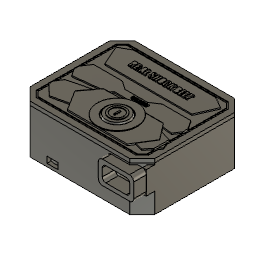
device_case (Autodesk Fusion 360 design; units mm, degrees)
part number: 2026-05-29-19-24-18-307
part number: 2026-05-29-19-24-19-033
part number: 2026-05-29-19-24-19-686
part number: 2026-05-29-19-24-22-511
part number: 2026-05-29-19-24-23-032
Autodesk Fusion 360 part; units mm, degrees
(part 1 of 2)
ref_plane "作業平面1" through (0, 0, 0) normal (0, 0, 1) x (1, 0, 0) in component "CASE_BASE_print"
sketch "スケッチ1" plane through (0, 0, 0) normal (0, 0, 1) x (1, 0, 0) in component "CASE_BASE_print"
  line L0 (-40, -42) -> (40, -42)
  line L1 (40, -42) -> (50, -32)
  line L2 (50, -32) -> (50, 32)
  line L3 (50, 32) -> (40, 42)
  line L4 (40, 42) -> (-40, 42)
  line L5 (-40, 42) -> (-50, 32)
  line L6 (-50, 32) -> (-50, -32)
  line L7 (-50, -32) -> (-40, -42)
extrude "押し出し1" add sketch "スケッチ1" along normal blind 36 makes body 1 in component "CASE_BASE_print"
ref_plane "作業平面2" through (0, 0, 2.4) normal (0, 0, 1) x (1, 0, 0) in component "CASE_BASE_print"
sketch "スケッチ2" plane through (0, 0, 2.4) normal (0, 0, 1) x (1, 0, 0) in component "CASE_BASE_print"
  line L0 (-40, -39.6) -> (40, -39.6)
  line L1 (40, -39.6) -> (47.6, -32)
  line L2 (47.6, -32) -> (47.6, 32)
  line L3 (47.6, 32) -> (40, 39.6)
  line L4 (40, 39.6) -> (-40, 39.6)
  line L5 (-40, 39.6) -> (-47.6, 32)
  line L6 (-47.6, 32) -> (-47.6, -32)
  line L7 (-47.6, -32) -> (-40, -39.6)
extrude "押し出し2" add sketch "スケッチ2" along normal blind 34.1 separate body makes body 2 in component "CASE_BASE_print"
ref_plane "作業平面3" through (0, 0, -0.5) normal (0, 0, 1) x (1, 0, 0) in component "CASE_BASE_print"
sketch "スケッチ3" plane through (0, 0, -0.5) normal (0, 0, 1) x (1, 0, 0) in component "CASE_BASE_print"
  circle A0 centre (-22, -14) radius 25.175
extrude "押し出し3" add sketch "スケッチ3" along normal blind 7.5 separate body makes body 3 in component "CASE_BASE_print"
combine "結合1" operation cut target body 1 tool bodies 2 3 in component "CASE_BASE_print"
ref_plane "作業平面4" through (0, 0, 0) normal (0, 0, 1) x (1, 0, 0) in component "CASE_BASE_print"
sketch "スケッチ4" plane through (0, 0, 0) normal (0, 0, 1) x (1, 0, 0) in component "CASE_BASE_print"
  circle A0 centre (-22, -14) radius 27.375
extrude "押し出し4" add sketch "スケッチ4" along normal blind 6.2 separate body makes body 4 in component "CASE_BASE_print"
ref_plane "作業平面5" through (0, 0, -0.2) normal (0, 0, 1) x (1, 0, 0) in component "CASE_BASE_print"
sketch "スケッチ5" plane through (0, 0, -0.2) normal (0, 0, 1) x (1, 0, 0) in component "CASE_BASE_print"
  circle A0 centre (-22, -14) radius 25.175
extrude "押し出し5" add sketch "スケッチ5" along normal blind 6.8 separate body makes body 5 in component "CASE_BASE_print"
combine "結合2" operation cut target body 4 tool bodies 5 in component "CASE_BASE_print"
combine "結合3" operation add target body 1 tool bodies 4 in component "CASE_BASE_print"
ref_plane "作業平面6" through (0, 0, 2.5) normal (0, 0, 1) x (1, 0, 0) in component "CASE_BASE_print"
sketch "スケッチ6" plane through (0, 0, 2.5) normal (0, 0, 1) x (1, 0, 0) in component "CASE_BASE_print"
  line L0 (-26.5, -42.5) -> (-17.5, -42.5)
  line L1 (-17.5, -42.5) -> (-17.5, -32)
  line L2 (-17.5, -32) -> (-26.5, -32)
  line L3 (-26.5, -32) -> (-26.5, -42.5)
extrude "押し出し6" add sketch "スケッチ6" along normal blind 5 separate body makes body 6 in component "CASE_BASE_print"
ref_plane "作業平面7" through (0, -42.7, 0) normal (0, 1, 0) x (0, 0, 1) in component "CASE_BASE_print"
sketch "スケッチ7" plane through (0, -42.7, 0) normal (0, 1, 0) x (1, 0, 0) in component "CASE_BASE_print"
  line L0 (27.8, 19.5) -> (44.2, 19.5)
  arc A0 (44.2, 19.5) -> (47, 22.3) centre (44.2, 22.3) ccw
  line L1 (47, 22.3) -> (47, 28.7)
  arc A1 (47, 28.7) -> (44.2, 31.5) centre (44.2, 28.7) ccw
  line L2 (44.2, 31.5) -> (27.8, 31.5)
  arc A2 (27.8, 31.5) -> (25, 28.7) centre (27.8, 28.7) ccw
  line L3 (25, 28.7) -> (25, 22.3)
  arc A3 (25, 22.3) -> (27.8, 19.5) centre (27.8, 22.3) ccw
extrude "押し出し7" add sketch "スケッチ7" along normal blind 7.1 separate body makes body 7 in component "CASE_BASE_print"
move_body "移動1" bodies 7 to x (1, 0, 0) y (0, 1, 0) z (0, 0, 1) at (0, 0, 51) in component "CASE_BASE_print"
combine "結合4" operation cut target body 1 tool bodies 6 7 in component "CASE_BASE_print"
ref_plane "作業平面8" through (0, -49, 0) normal (0, 1, 0) x (0, 0, 1) in component "CASE_BASE_print"
sketch "スケッチ8" plane through (0, -49, 0) normal (0, 1, 0) x (1, 0, 0) in component "CASE_BASE_print"
  line L0 (25.2, 16.3) -> (46.8, 16.3)
  arc A0 (46.8, 16.3) -> (50.2, 19.7) centre (46.8, 19.7) ccw
  line L1 (50.2, 19.7) -> (50.2, 31.3)
  arc A1 (50.2, 31.3) -> (46.8, 34.7) centre (46.8, 31.3) ccw
  line L2 (46.8, 34.7) -> (25.2, 34.7)
  arc A2 (25.2, 34.7) -> (21.8, 31.3) centre (25.2, 31.3) ccw
  line L3 (21.8, 31.3) -> (21.8, 19.7)
  arc A3 (21.8, 19.7) -> (25.2, 16.3) centre (25.2, 19.7) ccw
extrude "押し出し8" add sketch "スケッチ8" along normal blind 10.2 separate body makes body 8 in component "CASE_BASE_print"
move_body "移動2" bodies 8 to x (1, 0, 0) y (0, 1, 0) z (0, 0, 1) at (0, 0, 51) in component "CASE_BASE_print"
ref_plane "作業平面9" through (0, -49.2, 0) normal (0, 1, 0) x (0, 0, 1) in component "CASE_BASE_print"
sketch "スケッチ9" plane through (0, -49.2, 0) normal (0, 1, 0) x (1, 0, 0) in component "CASE_BASE_print"
  line L0 (27.8, 19.5) -> (44.2, 19.5)
  arc A0 (44.2, 19.5) -> (47, 22.3) centre (44.2, 22.3) ccw
  line L1 (47, 22.3) -> (47, 28.7)
  arc A1 (47, 28.7) -> (44.2, 31.5) centre (44.2, 28.7) ccw
  line L2 (44.2, 31.5) -> (27.8, 31.5)
  arc A2 (27.8, 31.5) -> (25, 28.7) centre (27.8, 28.7) ccw
  line L3 (25, 28.7) -> (25, 22.3)
  arc A3 (25, 22.3) -> (27.8, 19.5) centre (27.8, 22.3) ccw
extrude "押し出し9" add sketch "スケッチ9" along normal blind 10.6 separate body makes body 9 in component "CASE_BASE_print"
move_body "移動3" bodies 9 to x (1, 0, 0) y (0, 1, 0) z (0, 0, 1) at (0, 0, 51) in component "CASE_BASE_print"
combine "結合5" operation cut target body 8 tool bodies 9 in component "CASE_BASE_print"
combine "結合6" operation add target body 1 tool bodies 8 in component "CASE_BASE_print"
ref_plane "作業平面10" through (0, 0, 16.3) normal (0, 0, 1) x (1, 0, 0) in component "CASE_BASE_print"
sketch "スケッチ10" plane through (0, 0, 16.3) normal (0, 0, 1) x (1, 0, 0) in component "CASE_BASE_print"
  line L0 (47, -38.8) -> (50, -38.8)
  line L1 (50, -38.8) -> (50, -32)
  line L2 (50, -32) -> (47, -35)
  line L3 (47, -35) -> (47, -38.8)
extrude "押し出し10" add sketch "スケッチ10" along normal blind 18.4 separate body makes body 10 in component "CASE_BASE_print"
combine "結合7" operation add target body 1 tool bodies 10 in component "CASE_BASE_print"
ref_plane "作業平面11" through (0, 0, 2.4) normal (0, 0, 1) x (1, 0, 0) in component "CASE_BASE_print"
sketch "スケッチ11" plane through (0, 0, 2.4) normal (0, 0, 1) x (1, 0, 0) in component "CASE_BASE_print"
  circle A0 centre (12, -24) radius 2.9
extrude "押し出し11" add sketch "スケッチ11" along normal blind 15.1 separate body makes body 11 in component "CASE_BASE_print"
ref_plane "作業平面12" through (0, 0, 2.2) normal (0, 0, 1) x (1, 0, 0) in component "CASE_BASE_print"
sketch "スケッチ12" plane through (0, 0, 2.2) normal (0, 0, 1) x (1, 0, 0) in component "CASE_BASE_print"
  circle A0 centre (12, -24) radius 1.1
extrude "押し出し12" add sketch "スケッチ12" along normal blind 15.7 separate body makes body 12 in component "CASE_BASE_print"
combine "結合8" operation cut target body 11 tool bodies 12 in component "CASE_BASE_print"
ref_plane "作業平面13" through (0, 0, 2.4) normal (0, 0, 1) x (1, 0, 0) in component "CASE_BASE_print"
sketch "スケッチ13" plane through (0, 0, 2.4) normal (0, 0, 1) x (1, 0, 0) in component "CASE_BASE_print"
  circle A0 centre (42, -24) radius 2.9
extrude "押し出し13" add sketch "スケッチ13" along normal blind 15.1 separate body makes body 13 in component "CASE_BASE_print"
ref_plane "作業平面14" through (0, 0, 2.2) normal (0, 0, 1) x (1, 0, 0) in component "CASE_BASE_print"
sketch "スケッチ14" plane through (0, 0, 2.2) normal (0, 0, 1) x (1, 0, 0) in component "CASE_BASE_print"
  circle A0 centre (42, -24) radius 1.1
extrude "押し出し14" add sketch "スケッチ14" along normal blind 15.7 separate body makes body 14 in component "CASE_BASE_print"
combine "結合9" operation cut target body 13 tool bodies 14 in component "CASE_BASE_print"
ref_plane "作業平面15" through (0, 0, 2.4) normal (0, 0, 1) x (1, 0, 0) in component "CASE_BASE_print"
sketch "スケッチ15" plane through (0, 0, 2.4) normal (0, 0, 1) x (1, 0, 0) in component "CASE_BASE_print"
  circle A0 centre (-2, 28) radius 2.9
extrude "押し出し15" add sketch "スケッチ15" along normal blind 15.1 separate body makes body 15 in component "CASE_BASE_print"
ref_plane "作業平面16" through (0, 0, 2.2) normal (0, 0, 1) x (1, 0, 0) in component "CASE_BASE_print"
sketch "スケッチ16" plane through (0, 0, 2.2) normal (0, 0, 1) x (1, 0, 0) in component "CASE_BASE_print"
  circle A0 centre (-2, 28) radius 1.1
extrude "押し出し16" add sketch "スケッチ16" along normal blind 15.7 separate body makes body 16 in component "CASE_BASE_print"
combine "結合10" operation cut target body 15 tool bodies 16 in component "CASE_BASE_print"
ref_plane "作業平面17" through (0, 0, 2.4) normal (0, 0, 1) x (1, 0, 0) in component "CASE_BASE_print"
sketch "スケッチ17" plane through (0, 0, 2.4) normal (0, 0, 1) x (1, 0, 0) in component "CASE_BASE_print"
  circle A0 centre (42, 28) radius 2.9
extrude "押し出し17" add sketch "スケッチ17" along normal blind 15.1 separate body makes body 17 in component "CASE_BASE_print"
ref_plane "作業平面18" through (0, 0, 2.2) normal (0, 0, 1) x (1, 0, 0) in component "CASE_BASE_print"
sketch "スケッチ18" plane through (0, 0, 2.2) normal (0, 0, 1) x (1, 0, 0) in component "CASE_BASE_print"
  circle A0 centre (42, 28) radius 1.1
extrude "押し出し18" add sketch "スケッチ18" along normal blind 15.7 separate body makes body 18 in component "CASE_BASE_print"
combine "結合11" operation cut target body 17 tool bodies 18 in component "CASE_BASE_print"
combine "結合12" operation add target body 1 tool bodies 11 13 15 17 in component "CASE_BASE_print"
ref_plane "作業平面1" through (0, 0, 36) normal (0, 0, 1) x (1, 0, 0) in component "CASE_LID_print"
sketch "スケッチ1 (2)" plane through (0, 0, 36) normal (0, 0, 1) x (1, 0, 0) in component "CASE_LID_print"
  line L0 (-40, -42) -> (40, -42)
  line L1 (40, -42) -> (50, -32)
  line L2 (50, -32) -> (50, 32)
  line L3 (50, 32) -> (40, 42)
  line L4 (40, 42) -> (-40, 42)
  line L5 (-40, 42) -> (-50, 32)
  line L6 (-50, 32) -> (-50, -32)
  line L7 (-50, -32) -> (-40, -42)
extrude "押し出し1'" add sketch "スケッチ1 (2)" along normal blind 3 separate body makes body 19 in component "CASE_LID_print"
ref_plane "作業平面2" through (0, 0, 33) normal (0, 0, 1) x (1, 0, 0) in component "CASE_LID_print"
sketch "スケッチ2 (2)" plane through (0, 0, 33) normal (0, 0, 1) x (1, 0, 0) in component "CASE_LID_print"
  line L0 (-40, -39.25) -> (40, -39.25)
  line L1 (40, -39.25) -> (47.25, -32)
  line L2 (47.25, -32) -> (47.25, 32)
  line L3 (47.25, 32) -> (40, 39.25)
  line L4 (40, 39.25) -> (-40, 39.25)
  line L5 (-40, 39.25) -> (-47.25, 32)
  line L6 (-47.25, 32) -> (-47.25, -32)
  line L7 (-47.25, -32) -> (-40, -39.25)
extrude "押し出し2'" add sketch "スケッチ2 (2)" along normal blind 3 separate body makes body 20 in component "CASE_LID_print"
ref_plane "作業平面3" through (0, 0, 32.8) normal (0, 0, 1) x (1, 0, 0) in component "CASE_LID_print"
sketch "スケッチ3 (2)" plane through (0, 0, 32.8) normal (0, 0, 1) x (1, 0, 0) in component "CASE_LID_print"
  line L0 (-40, -37.45) -> (40, -37.45)
  line L1 (40, -37.45) -> (45.45, -32)
  line L2 (45.45, -32) -> (45.45, 32)
  line L3 (45.45, 32) -> (40, 37.45)
  line L4 (40, 37.45) -> (-40, 37.45)
  line L5 (-40, 37.45) -> (-45.45, 32)
  line L6 (-45.45, 32) -> (-45.45, -32)
  line L7 (-45.45, -32) -> (-40, -37.45)
extrude "押し出し3'" add sketch "スケッチ3 (2)" along normal blind 3.4 separate body makes body 21 in component "CASE_LID_print"
combine "結合1'" operation cut target body 20 tool bodies 21 in component "CASE_LID_print"
combine "結合2'" operation add target body 19 tool bodies 20 in component "CASE_LID_print"
ref_plane "作業平面4" through (0, 0, 32.7) normal (0, 0, 1) x (1, 0, 0) in component "CASE_LID_print"
sketch "スケッチ4 (2)" plane through (0, 0, 32.7) normal (0, 0, 1) x (1, 0, 0) in component "CASE_LID_print"
  circle A0 centre (6, -18) radius 5.25
extrude "押し出し4'" add sketch "スケッチ4 (2)" along normal blind 6.6 separate body makes body 22 in component "CASE_LID_print"
ref_plane "作業平面5" through (0, 0, 35) normal (0, 0, 1) x (1, 0, 0) in component "CASE_LID_print"
sketch "スケッチ5 (2)" plane through (0, 0, 35) normal (0, 0, 1) x (1, 0, 0) in component "CASE_LID_print"
  circle A0 centre (6, -18) radius 9.9
extrude "押し出し5'" add sketch "スケッチ5 (2)" along normal blind 4.3 separate body makes body 23 in component "CASE_LID_print"
combine "結合3'" operation cut target body 19 tool bodies 22 23 in component "CASE_LID_print"
ref_plane "作業平面6" through (0, 0, 26) normal (0, 0, 1) x (1, 0, 0) in component "CASE_LID_print"
sketch "スケッチ6 (2)" plane through (0, 0, 26) normal (0, 0, 1) x (1, 0, 0) in component "CASE_LID_print"
  circle A0 centre (6, -18) radius 11.5
extrude "押し出し6'" add sketch "スケッチ6 (2)" along normal blind 10.6 separate body makes body 24 in component "CASE_LID_print"
ref_plane "作業平面7" through (0, 0, 25.8) normal (0, 0, 1) x (1, 0, 0) in component "CASE_LID_print"
sketch "スケッチ7 (2)" plane through (0, 0, 25.8) normal (0, 0, 1) x (1, 0, 0) in component "CASE_LID_print"
  circle A0 centre (6, -18) radius 5.25
extrude "押し出し7'" add sketch "スケッチ7 (2)" along normal blind 11.1 separate body makes body 25 in component "CASE_LID_print"
combine "結合4'" operation cut target body 24 tool bodies 25 in component "CASE_LID_print"
combine "結合5'" operation add target body 19 tool bodies 24 in component "CASE_LID_print"
ref_plane "作業平面8" through (0, 0, 38.95) normal (0, 0, 1) x (1, 0, 0) in component "CASE_LID_print"
sketch "スケッチ8 (2)" plane through (0, 0, 38.95) normal (0, 0, 1) x (1, 0, 0) in component "CASE_LID_print"
  line L0 (-42, 29) -> (-33, 34)
  line L1 (-33, 34) -> (33, 34)
  line L2 (33, 34) -> (42, 29)
  line L3 (42, 29) -> (35, 13)
  line L4 (35, 13) -> (-35, 13)
  line L5 (-35, 13) -> (-42, 29)
extrude "押し出し8'" add sketch "スケッチ8 (2)" along normal blind 1 separate body makes body 26 in component "CASE_LID_print"
ref_plane "作業平面9" through (0, 0, 38.95) normal (0, 0, 1) x (1, 0, 0) in component "CASE_LID_print"
sketch "スケッチ9 (2)" plane through (0, 0, 38.95) normal (0, 0, 1) x (1, 0, 0) in component "CASE_LID_print"
  line L0 (-39, 8) -> (-16, 8)
  line L1 (-16, 8) -> (-8, 2.5)
  line L2 (-8, 2.5) -> (-14, -5.5)
  line L3 (-14, -5.5) -> (-40, -8.5)
  line L4 (-40, -8.5) -> (-45, -1)
  line L5 (-45, -1) -> (-39, 8)
extrude "押し出し9'" add sketch "スケッチ9 (2)" along normal blind 1 separate body makes body 27 in component "CASE_LID_print"
ref_plane "作業平面10" through (0, 0, 38.95) normal (0, 0, 1) x (1, 0, 0) in component "CASE_LID_print"
sketch "スケッチ10 (2)" plane through (0, 0, 38.95) normal (0, 0, 1) x (1, 0, 0) in component "CASE_LID_print"
  line L0 (39, 8) -> (16, 8)
  line L1 (16, 8) -> (8, 2.5)
  line L2 (8, 2.5) -> (14, -5.5)
  line L3 (14, -5.5) -> (40, -8.5)
  line L4 (40, -8.5) -> (45, -1)
  line L5 (45, -1) -> (39, 8)
extrude "押し出し10'" add sketch "スケッチ10 (2)" along normal blind 1 separate body makes body 28 in component "CASE_LID_print"
ref_plane "作業平面11" through (0, 0, 38.95) normal (0, 0, 1) x (1, 0, 0) in component "CASE_LID_print"
sketch "スケッチ11 (2)" plane through (0, 0, 38.95) normal (0, 0, 1) x (1, 0, 0) in component "CASE_LID_print"
  line L0 (-40, -14) -> (-20, -9)
  line L1 (-20, -9) -> (-7, -14)
  line L2 (-7, -14) -> (-15, -27)
  line L3 (-15, -27) -> (-35, -31.5)
  line L4 (-35, -31.5) -> (-45, -22)
  line L5 (-45, -22) -> (-40, -14)
extrude "押し出し11'" add sketch "スケッチ11 (2)" along normal blind 1 separate body makes body 29 in component "CASE_LID_print"
ref_plane "作業平面12" through (0, 0, 38.95) normal (0, 0, 1) x (1, 0, 0) in component "CASE_LID_print"
sketch "スケッチ12 (2)" plane through (0, 0, 38.95) normal (0, 0, 1) x (1, 0, 0) in component "CASE_LID_print"
  line L0 (44, -14) -> (26, -9)
  line L1 (26, -9) -> (13, -14)
  line L2 (13, -14) -> (21, -27)
  line L3 (21, -27) -> (39, -31.5)
  line L4 (39, -31.5) -> (47, -22)
  line L5 (47, -22) -> (44, -14)
extrude "押し出し12'" add sketch "スケッチ12 (2)" along normal blind 1 separate body makes body 30 in component "CASE_LID_print"
ref_plane "作業平面13" through (0, 0, 38.95) normal (0, 0, 1) x (1, 0, 0) in component "CASE_LID_print"
sketch "スケッチ13 (2)" plane through (0, 0, 38.95) normal (0, 0, 1) x (1, 0, 0) in component "CASE_LID_print"
  line L0 (-18, -5) -> (30, -5)
  line L1 (30, -5) -> (40, -18)
  line L2 (40, -18) -> (30, -34)
  line L3 (30, -34) -> (-18, -34)
  line L4 (-18, -34) -> (-28, -18)
  line L5 (-28, -18) -> (-18, -5)
extrude "押し出し13'" add sketch "スケッチ13 (2)" along normal blind 1.2 separate body makes body 31 in component "CASE_LID_print"
ref_plane "作業平面14" through (0, 0, 38.95) normal (0, 0, 1) x (1, 0, 0) in component "CASE_LID_print"
sketch "スケッチ14 (2)" plane through (0, 0, 38.95) normal (0, 0, 1) x (1, 0, 0) in component "CASE_LID_print"
  line L0 (-13, -2.6) -> (25, -2.6)
  line L1 (25, -2.6) -> (28, 0.5)
  line L2 (28, 0.5) -> (24, 3.3)
  line L3 (24, 3.3) -> (-12, 3.3)
  line L4 (-12, 3.3) -> (-16, 0.5)
  line L5 (-16, 0.5) -> (-13, -2.6)
extrude "押し出し14'" add sketch "スケッチ14 (2)" along normal blind 1 separate body makes body 32 in component "CASE_LID_print"
combine "結合6'" operation add target body 19 tool bodies 26 27 28 29 30 31 32 in component "CASE_LID_print"
ref_plane "作業平面15" through (0, 0, 39.9) normal (0, 0, 1) x (1, 0, 0) in component "CASE_LID_print"
sketch "スケッチ15 (2)" plane through (0, 0, 39.9) normal (0, 0, 1) x (1, 0, 0) in component "CASE_LID_print"
  line L0 (0.01, 25.6699) -> (1.0286, 25.6699)
  spline S0 degree 3 poles (1.0286, 25.6699) (1.3136, 25.6712) (1.7747, 25.6732) (2.2316, 25.6139) (2.406, 25.5913) knots 0 0 0 0 0.085386 0.138098 0.138098 0.138098 0.138098
  spline S1 degree 3 poles (2.406, 25.5913) (2.5217, 25.5539) (2.7574, 25.4777) (2.9141, 25.2857) (2.9939, 25.188) knots 0 0 0 0 0.03568 0.072659 0.072659 0.072659 0.072659
  spline S2 degree 3 poles (2.9939, 25.188) (3.0603, 25.0509) (3.2169, 24.7278) (3.2207, 24.367) (3.2229, 24.1592) knots 0 0 0 0 0.045177 0.106541 0.106541 0.106541 0.106541
  spline S3 degree 3 poles (3.2229, 24.1592) (3.2243, 23.9759) (3.2267, 23.6744) (3.1086, 23.399) (3.0622, 23.291) knots 0 0 0 0 0.054153 0.089108 0.089108 0.089108 0.089108
  spline S4 degree 3 poles (3.0622, 23.291) (2.9864, 23.2238) (2.8077, 23.0654) (2.568, 23.0394) (2.4299, 23.0244) knots 0 0 0 0 0.029736 0.070118 0.070118 0.070118 0.070118
  spline S5 degree 3 poles (2.4299, 23.0244) (2.5541, 22.9928) (2.7668, 22.9388) (2.9344, 22.7989) (3.0041, 22.7407) knots 0 0 0 0 0.037806 0.064758 0.064758 0.064758 0.064758
  spline S6 degree 3 poles (3.0041, 22.7407) (3.0476, 22.6858) (3.1264, 22.5863) (3.1671, 22.4664) (3.1853, 22.4126) knots 0 0 0 0 0.020812 0.037727 0.037727 0.037727 0.037727
  spline S7 degree 3 poles (3.1853, 22.4126) (3.196, 22.3201) (3.2275, 22.0489) (3.2247, 21.7757) (3.2229, 21.5957) knots 0 0 0 0 0.027914 0.08184 0.08184 0.08184 0.08184
  line L1 (3.2229, 21.5957) -> (3.2229, 20.1362)
  line L2 (3.2229, 20.1362) -> (1.8865, 20.1362)
  line L3 (1.8865, 20.1362) -> (1.8865, 21.9751)
  spline S8 degree 3 poles (1.8865, 21.9751) (1.8891, 22.0964) (1.8931, 22.2844) (1.8352, 22.4623) (1.8147, 22.5254) knots 0 0 0 0 0.036019 0.05582 0.05582 0.05582 0.05582
  spline S9 degree 3 poles (1.8147, 22.5254) (1.7742, 22.5559) (1.668, 22.6359) (1.5327, 22.6331) (1.449, 22.6313) knots 0 0 0 0 0.014864 0.039021 0.039021 0.039021 0.039021
  line L4 (1.449, 22.6313) -> (1.449, 20.1362)
  line L5 (1.449, 20.1362) -> (0.01, 20.1362)
  line L6 (0.01, 20.1362) -> (0.01, 25.6699)
  line L7 (1.449, 24.7231) -> (1.449, 23.4927)
  spline S10 degree 3 poles (1.449, 23.4927) (1.5188, 23.4926) (1.6363, 23.4925) (1.7438, 23.5388) (1.7873, 23.5576) knots 0 0 0 0 0.020657 0.034769 0.034769 0.034769 0.034769
  spline S11 degree 3 poles (1.7873, 23.5576) (1.8157, 23.6041) (1.8956, 23.7352) (1.8901, 23.8911) (1.8865, 23.9917) knots 0 0 0 0 0.01609 0.045334 0.045334 0.045334 0.045334
  line L8 (1.8865, 23.9917) -> (1.8865, 24.2959)
  spline S12 degree 3 poles (1.8865, 24.2959) (1.8869, 24.3712) (1.8875, 24.4968) (1.8184, 24.5999) (1.7908, 24.6411) knots 0 0 0 0 0.021921 0.036536 0.036536 0.036536 0.036536
  spline S13 degree 3 poles (1.7908, 24.6411) (1.7478, 24.6648) (1.6423, 24.723) (1.5209, 24.7231) (1.449, 24.7231) knots 0 0 0 0 0.014526 0.035647 0.035647 0.035647 0.035647
  line L9 (3.78, 25.6699) -> (6.1794, 25.6699)
  line L10 (6.1794, 25.6699) -> (6.1794, 24.5625)
  line L11 (6.1794, 24.5625) -> (5.219, 24.5625)
  line L12 (5.219, 24.5625) -> (5.219, 23.5132)
  line L13 (5.219, 23.5132) -> (6.1179, 23.5132)
  line L14 (6.1179, 23.5132) -> (6.1179, 22.4604)
  line L15 (6.1179, 22.4604) -> (5.219, 22.4604)
  line L16 (5.219, 22.4604) -> (5.219, 21.2436)
  line L17 (5.219, 21.2436) -> (6.2751, 21.2436)
  line L18 (6.2751, 21.2436) -> (6.2751, 20.1362)
  line L19 (6.2751, 20.1362) -> (3.78, 20.1362)
  line L20 (3.78, 20.1362) -> (3.78, 25.6699)
  line L21 (7.6902, 23.7388) -> (7.6902, 22.6142)
  line L22 (7.6902, 22.6142) -> (6.6477, 22.6142)
  line L23 (6.6477, 22.6142) -> (6.6477, 23.7388)
  line L24 (6.6477, 23.7388) -> (7.6902, 23.7388)
  line L25 (7.6902, 21.2641) -> (7.6902, 20.1362)
  line L26 (7.6902, 20.1362) -> (6.6477, 20.1362)
  line L27 (6.6477, 20.1362) -> (6.6477, 21.2641)
  line L28 (6.6477, 21.2641) -> (7.6902, 21.2641)
  line L29 (10.5886, 25.6699) -> (11.4123, 20.1362)
  line L30 (11.4123, 20.1362) -> (9.9392, 20.1362)
  line L31 (9.9392, 20.1362) -> (9.8674, 21.1308)
  line L32 (9.8674, 21.1308) -> (9.3513, 21.1308)
  line L33 (9.3513, 21.1308) -> (9.2659, 20.1362)
  line L34 (9.2659, 20.1362) -> (7.7756, 20.1362)
  line L35 (7.7756, 20.1362) -> (8.5071, 25.6699)
  line L36 (8.5071, 25.6699) -> (10.5886, 25.6699)
  spline S14 degree 3 poles (9.8264, 22.1118) (9.7885, 22.4617) (9.7049, 23.2343) (9.642, 24.0089) (9.6077, 24.4326) knots 0 0 0 0 0.105585 0.233118 0.233118 0.233118 0.233118
  spline S15 degree 3 poles (9.6077, 24.4326) (9.5446, 23.9753) (9.4382, 23.2035) (9.3643, 22.4279) (9.3342, 22.1118) knots 0 0 0 0 0.138462 0.233708 0.233708 0.233708 0.233708
  line L37 (9.3342, 22.1118) -> (9.8264, 22.1118)
  line L38 (13.0974, 25.6699) -> (13.0974, 21.2436)
  line L39 (13.0974, 21.2436) -> (13.9724, 21.2436)
  line L40 (13.9724, 21.2436) -> (13.9724, 20.1362)
  line L41 (13.9724, 20.1362) -> (11.6584, 20.1362)
  line L42 (11.6584, 20.1362) -> (11.6584, 25.6699)
  line L43 (11.6584, 25.6699) -> (13.0974, 25.6699)
  line L44 (18.6037, 23.9951) -> (17.2673, 23.9951)
  line L45 (17.2673, 23.9951) -> (17.2673, 24.4053)
  spline S16 degree 3 poles (17.2673, 24.4053) (17.2687, 24.4846) (17.2709, 24.6098) (17.2308, 24.7277) (17.2161, 24.771) knots 0 0 0 0 0.023533 0.037161 0.037161 0.037161 0.037161
  spline S17 degree 3 poles (17.2161, 24.771) (17.1948, 24.7939) (17.1491, 24.8433) (17.0814, 24.8474) (17.0452, 24.8496) knots 0 0 0 0 0.009027 0.019468 0.019468 0.019468 0.019468
  spline S18 degree 3 poles (17.0452, 24.8496) (17.0045, 24.8453) (16.924, 24.8369) (16.8725, 24.7745) (16.8469, 24.7436) knots 0 0 0 0 0.011753 0.023297 0.023297 0.023297 0.023297
  spline S19 degree 3 poles (16.8469, 24.7436) (16.8281, 24.6998) (16.7842, 24.5976) (16.7828, 24.486) (16.782, 24.4223) knots 0 0 0 0 0.014192 0.033061 0.033061 0.033061 0.033061
  spline S20 degree 3 poles (16.782, 24.4223) (16.7829, 24.3404) (16.7845, 24.1968) (16.8353, 24.0629) (16.8572, 24.0054) knots 0 0 0 0 0.02434 0.042662 0.042662 0.042662 0.042662
  spline S21 degree 3 poles (16.8572, 24.0054) (16.9009, 23.9513) (17.0134, 23.8123) (17.1688, 23.7221) (17.2639, 23.667) knots 0 0 0 0 0.0207 0.053288 0.053288 0.053288 0.053288
  spline S22 degree 3 poles (17.2639, 23.667) (17.5361, 23.5077) (17.9812, 23.2473) (18.336, 22.8751) (18.4739, 22.7304) knots 0 0 0 0 0.093944 0.153645 0.153645 0.153645 0.153645
  spline S23 degree 3 poles (18.4739, 22.7304) (18.5462, 22.5736) (18.7178, 22.2013) (18.7213, 21.7895) (18.7234, 21.5513) knots 0 0 0 0 0.051301 0.121732 0.121732 0.121732 0.121732
  spline S24 degree 3 poles (18.7234, 21.5513) (18.7223, 21.3782) (18.7205, 21.0796) (18.6239, 20.798) (18.5832, 20.6797) knots 0 0 0 0 0.051474 0.088788 0.088788 0.088788 0.088788
  spline S25 degree 3 poles (18.5832, 20.6797) (18.5216, 20.5875) (18.3857, 20.3845) (18.1686, 20.2704) (18.05, 20.208) knots 0 0 0 0 0.032751 0.072191 0.072191 0.072191 0.072191
  spline S26 degree 3 poles (18.05, 20.208) (17.9087, 20.1532) (17.612, 20.0382) (17.2938, 20.0262) (17.1272, 20.02) knots 0 0 0 0 0.045153 0.094766 0.094766 0.094766 0.094766
  spline S27 degree 3 poles (17.1272, 20.02) (16.946, 20.0269) (16.603, 20.0399) (16.288, 20.175) (16.1394, 20.2388) knots 0 0 0 0 0.053855 0.101943 0.101943 0.101943 0.101943
  spline S28 degree 3 poles (16.1394, 20.2388) (16.0172, 20.3124) (15.7883, 20.4503) (15.6641, 20.686) (15.6062, 20.7959) knots 0 0 0 0 0.041854 0.07843 0.07843 0.07843 0.07843
  spline S29 degree 3 poles (15.6062, 20.7959) (15.5695, 20.9316) (15.4845, 21.2456) (15.4815, 21.5713) (15.4797, 21.7563) knots 0 0 0 0 0.042015 0.09722 0.09722 0.09722 0.09722
  line L46 (15.4797, 21.7563) -> (15.4797, 22.1186)
  line L47 (15.4797, 22.1186) -> (16.8162, 22.1186)
  line L48 (16.8162, 22.1186) -> (16.8162, 21.4453)
  spline S30 degree 3 poles (16.8162, 21.4453) (16.8148, 21.3591) (16.8127, 21.2225) (16.8551, 21.0932) (16.8708, 21.0454) knots 0 0 0 0 0.025586 0.040598 0.040598 0.040598 0.040598
  spline S31 degree 3 poles (16.8708, 21.0454) (16.8956, 21.0195) (16.9501, 20.9627) (17.0293, 20.9587) (17.0725, 20.9565) knots 0 0 0 0 0.010372 0.022791 0.022791 0.022791 0.022791
  spline S32 degree 3 poles (17.0725, 20.9565) (17.1169, 20.9607) (17.2035, 20.9689) (17.2579, 21.0364) (17.2844, 21.0693) knots 0 0 0 0 0.01279 0.024936 0.024936 0.024936 0.024936
  spline S33 degree 3 poles (17.2844, 21.0693) (17.3053, 21.1154) (17.3533, 21.2214) (17.3551, 21.3382) (17.3562, 21.4043) knots 0 0 0 0 0.015012 0.034577 0.034577 0.034577 0.034577
  spline S34 degree 3 poles (17.3562, 21.4043) (17.3579, 21.5422) (17.3607, 21.7669) (17.2613, 21.9664) (17.2229, 22.0434) knots 0 0 0 0 0.040555 0.066092 0.066092 0.066092 0.066092
  spline S35 degree 3 poles (17.2229, 22.0434) (17.1451, 22.1119) (16.9345, 22.2973) (16.6985, 22.4497) (16.5496, 22.5459) knots 0 0 0 0 0.03104 0.08411 0.08411 0.08411 0.08411
  spline S36 degree 3 poles (16.5496, 22.5459) (16.3987, 22.6452) (16.1537, 22.8064) (15.9261, 22.9911) (15.8386, 23.062) knots 0 0 0 0 0.054135 0.087898 0.087898 0.087898 0.087898
  spline S37 degree 3 poles (15.8386, 23.062) (15.7818, 23.1235) (15.6602, 23.2551) (15.5871, 23.419) (15.5481, 23.5063) knots 0 0 0 0 0.024934 0.053406 0.053406 0.053406 0.053406
  spline S38 degree 3 poles (15.5481, 23.5063) (15.5153, 23.6132) (15.4429, 23.849) (15.438, 24.096) (15.4353, 24.2309) knots 0 0 0 0 0.033389 0.073649 0.073649 0.073649 0.073649
  spline S39 degree 3 poles (15.4353, 24.2309) (15.4364, 24.4167) (15.4383, 24.7366) (15.5494, 25.0354) (15.5959, 25.1606) knots 0 0 0 0 0.055176 0.094982 0.094982 0.094982 0.094982
  spline S40 degree 3 poles (15.5959, 25.1606) (15.6614, 25.2543) (15.7985, 25.4504) (16.0112, 25.5609) (16.1223, 25.6186) knots 0 0 0 0 0.033764 0.070701 0.070701 0.070701 0.070701
  spline S41 degree 3 poles (16.1223, 25.6186) (16.2542, 25.6674) (16.5363, 25.7717) (16.8372, 25.7811) (16.9973, 25.7861) knots 0 0 0 0 0.041917 0.08961 0.08961 0.08961 0.08961
  spline S42 degree 3 poles (16.9973, 25.7861) (17.1721, 25.7808) (17.4999, 25.7708) (17.8074, 25.6577) (17.9509, 25.605) knots 0 0 0 0 0.052065 0.097631 0.097631 0.097631 0.097631
  spline S43 degree 3 poles (17.9509, 25.605) (18.0691, 25.546) (18.2844, 25.4385) (18.415, 25.2376) (18.4739, 25.147) knots 0 0 0 0 0.038766 0.070641 0.070641 0.070641 0.070641
  spline S44 degree 3 poles (18.4739, 25.147) (18.5114, 25.0244) (18.6043, 24.7213) (18.604, 24.4033) (18.6037, 24.2138) knots 0 0 0 0 0.03826 0.094665 0.094665 0.094665 0.094665
  line L49 (18.6037, 24.2138) -> (18.6037, 23.9951)
  line L50 (22.4831, 25.6699) -> (22.4831, 20.1362)
  line L51 (22.4831, 20.1362) -> (21.0442, 20.1362)
  line L52 (21.0442, 20.1362) -> (21.0442, 22.4604)
  line L53 (21.0442, 22.4604) -> (20.6135, 22.4604)
  line L54 (20.6135, 22.4604) -> (20.6135, 20.1362)
  line L55 (20.6135, 20.1362) -> (19.1746, 20.1362)
  line L56 (19.1746, 20.1362) -> (19.1746, 25.6699)
  line L57 (19.1746, 25.6699) -> (20.6135, 25.6699)
  line L58 (20.6135, 25.6699) -> (20.6135, 23.6909)
  line L59 (20.6135, 23.6909) -> (21.0442, 23.6909)
  line L60 (21.0442, 23.6909) -> (21.0442, 25.6699)
  line L61 (21.0442, 25.6699) -> (22.4831, 25.6699)
  spline S45 degree 3 poles (26.3489, 22.4297) (26.3491, 22.192) (26.3495, 21.7972) (26.3197, 21.4036) (26.3079, 21.2471) knots 0 0 0 0 0.071272 0.11837 0.11837 0.11837 0.11837
  spline S46 degree 3 poles (26.3079, 21.2471) (26.288, 21.1341) (26.2481, 20.907) (26.1241, 20.7125) (26.0618, 20.6147) knots 0 0 0 0 0.03403 0.068449 0.068449 0.068449 0.068449
  spline S47 degree 3 poles (26.0618, 20.6147) (25.986, 20.524) (25.831, 20.3385) (25.615, 20.2295) (25.5046, 20.1738) knots 0 0 0 0 0.035055 0.07172 0.07172 0.07172 0.07172
  spline S48 degree 3 poles (25.5046, 20.1738) (25.3788, 20.129) (25.1137, 20.0345) (24.8322, 20.025) (24.6843, 20.02) knots 0 0 0 0 0.039818 0.083907 0.083907 0.083907 0.083907
  spline S49 degree 3 poles (24.6843, 20.02) (24.5423, 20.025) (24.2687, 20.0347) (24.0093, 20.1217) (23.8845, 20.1636) knots 0 0 0 0 0.042364 0.081638 0.081638 0.081638 0.081638
  spline S50 degree 3 poles (23.8845, 20.1636) (23.7734, 20.2178) (23.5542, 20.3249) (23.3954, 20.5099) (23.3171, 20.6011) knots 0 0 0 0 0.036672 0.072322 0.072322 0.072322 0.072322
  spline S51 degree 3 poles (23.3171, 20.6011) (23.2527, 20.6993) (23.1255, 20.8932) (23.0822, 21.121) (23.0608, 21.2334) knots 0 0 0 0 0.034859 0.068828 0.068828 0.068828 0.068828
  spline S52 degree 3 poles (23.0608, 21.2334) (23.0489, 21.39) (23.0189, 21.7881) (23.0194, 22.1874) (23.0198, 22.4297) knots 0 0 0 0 0.047098 0.119737 0.119737 0.119737 0.119737
  line L62 (23.0198, 22.4297) -> (23.0198, 23.3764)
  spline S53 degree 3 poles (23.0198, 23.3764) (23.0195, 23.6138) (23.0192, 24.0074) (23.0465, 24.3999) (23.0574, 24.5556) knots 0 0 0 0 0.071185 0.118011 0.118011 0.118011 0.118011
  spline S54 degree 3 poles (23.0574, 24.5556) (23.0779, 24.6694) (23.1191, 24.8971) (23.2419, 25.0932) (23.3035, 25.1914) knots 0 0 0 0 0.03432 0.068732 0.068732 0.068732 0.068732
  spline S55 degree 3 poles (23.3035, 25.1914) (23.3801, 25.282) (23.5367, 25.4672) (23.7534, 25.5765) (23.864, 25.6323) knots 0 0 0 0 0.035232 0.071972 0.071972 0.071972 0.071972
  spline S56 degree 3 poles (23.864, 25.6323) (23.9898, 25.6771) (24.2549, 25.7716) (24.5364, 25.7811) (24.6843, 25.7861) knots 0 0 0 0 0.039818 0.083907 0.083907 0.083907 0.083907
  spline S57 degree 3 poles (24.6843, 25.7861) (24.8261, 25.781) (25.0989, 25.7712) (25.3568, 25.682) (25.4807, 25.6391) knots 0 0 0 0 0.042286 0.081384 0.081384 0.081384 0.081384
  spline S58 degree 3 poles (25.4807, 25.6391) (25.5928, 25.5859) (25.8135, 25.4811) (25.973, 25.2961) (26.0515, 25.2051) knots 0 0 0 0 0.036768 0.072417 0.072417 0.072417 0.072417
  spline S59 degree 3 poles (26.0515, 25.2051) (26.1159, 25.1068) (26.2431, 24.9129) (26.2865, 24.6851) (26.3079, 24.5727) knots 0 0 0 0 0.034859 0.068827 0.068827 0.068827 0.068827
  spline S60 degree 3 poles (26.3079, 24.5727) (26.3197, 24.4161) (26.3498, 24.018) (26.3492, 23.6187) (26.3489, 23.3764) knots 0 0 0 0 0.047098 0.119737 0.119737 0.119737 0.119737
  line L63 (26.3489, 23.3764) -> (26.3489, 22.4297)
  spline S61 degree 3 poles (24.9099, 24.248) (24.9113, 24.354) (24.9134, 24.5199) (24.8782, 24.6817) (24.8655, 24.7402) knots 0 0 0 0 0.031636 0.049551 0.049551 0.049551 0.049551
  spline S62 degree 3 poles (24.8655, 24.7402) (24.8471, 24.7721) (24.8085, 24.8388) (24.7314, 24.8459) (24.6912, 24.8496) knots 0 0 0 0 0.01041 0.021767 0.021767 0.021767 0.021767
  spline S63 degree 3 poles (24.6912, 24.8496) (24.6558, 24.8461) (24.5861, 24.8391) (24.5397, 24.7866) (24.5168, 24.7607) knots 0 0 0 0 0.010241 0.020226 0.020226 0.020226 0.020226
  spline S64 degree 3 poles (24.5168, 24.7607) (24.5003, 24.7041) (24.4515, 24.5375) (24.4559, 24.3631) (24.4587, 24.248) knots 0 0 0 0 0.017637 0.051847 0.051847 0.051847 0.051847
  line L64 (24.4587, 24.248) -> (24.4587, 21.664)
  spline S65 degree 3 poles (24.4587, 21.664) (24.4571, 21.5338) (24.4546, 21.3343) (24.4856, 21.1376) (24.4963, 21.0693) knots 0 0 0 0 0.038976 0.059677 0.059677 0.059677 0.059677
  spline S66 degree 3 poles (24.4963, 21.0693) (24.5156, 21.0364) (24.5564, 20.9666) (24.6378, 20.96) (24.6809, 20.9565) knots 0 0 0 0 0.01077 0.022894 0.022894 0.022894 0.022894
  spline S67 degree 3 poles (24.6809, 20.9565) (24.7253, 20.9614) (24.8118, 20.9708) (24.8502, 21.0485) (24.8689, 21.0864) knots 0 0 0 0 0.012478 0.02433 0.02433 0.02433 0.02433
  spline S68 degree 3 poles (24.8689, 21.0864) (24.8806, 21.1595) (24.9135, 21.3641) (24.9113, 21.5716) (24.9099, 21.7051) knots 0 0 0 0 0.022175 0.062093 0.062093 0.062093 0.062093
  line L65 (24.9099, 21.7051) -> (24.9099, 24.248)
  line L66 (30.2454, 23.2568) -> (28.8064, 23.2568)
  line L67 (28.8064, 23.2568) -> (28.8064, 24.2207)
  spline S69 degree 3 poles (28.8064, 24.2207) (28.8082, 24.335) (28.8111, 24.5115) (28.7722, 24.6832) (28.7585, 24.7436) knots 0 0 0 0 0.034115 0.052666 0.052666 0.052666 0.052666
  spline S70 degree 3 poles (28.7585, 24.7436) (28.7368, 24.7745) (28.6884, 24.843) (28.6036, 24.8472) (28.5569, 24.8496) knots 0 0 0 0 0.010766 0.023938 0.023938 0.023938 0.023938
  spline S71 degree 3 poles (28.5569, 24.8496) (28.504, 24.8465) (28.4069, 24.8408) (28.3549, 24.7599) (28.3313, 24.7231) knots 0 0 0 0 0.014866 0.027295 0.027295 0.027295 0.027295
  spline S72 degree 3 poles (28.3313, 24.7231) (28.3175, 24.6567) (28.2803, 24.4766) (28.2822, 24.2924) (28.2834, 24.1763) knots 0 0 0 0 0.020315 0.055028 0.055028 0.055028 0.055028
  line L68 (28.2834, 24.1763) -> (28.2834, 21.6059)
  spline S73 degree 3 poles (28.2834, 21.6059) (28.2823, 21.4943) (28.2805, 21.3169) (28.3175, 21.1437) (28.3313, 21.0796) knots 0 0 0 0 0.033347 0.052989 0.052989 0.052989 0.052989
  spline S74 degree 3 poles (28.3313, 21.0796) (28.3541, 21.0437) (28.4037, 20.9661) (28.4966, 20.9599) (28.5466, 20.9565) knots 0 0 0 0 0.012068 0.026165 0.026165 0.026165 0.026165
  spline S75 degree 3 poles (28.5466, 20.9565) (28.5948, 20.9602) (28.6855, 20.9671) (28.7329, 21.0437) (28.7551, 21.0796) knots 0 0 0 0 0.013597 0.025556 0.025556 0.025556 0.025556
  spline S76 degree 3 poles (28.7551, 21.0796) (28.7698, 21.148) (28.8106, 21.3379) (28.808, 21.5327) (28.8064, 21.6572) knots 0 0 0 0 0.020949 0.058142 0.058142 0.058142 0.058142
  line L69 (28.8064, 21.6572) -> (28.8064, 22.3511)
  line L70 (28.8064, 22.3511) -> (30.2454, 22.3511)
  line L71 (30.2454, 22.3511) -> (30.2454, 22.1357)
  spline S77 degree 3 poles (30.2454, 22.1357) (30.2457, 21.8901) (30.2464, 21.4797) (30.1579, 21.0796) (30.1223, 20.9189) knots 0 0 0 0 0.07338 0.122617 0.122617 0.122617 0.122617
  spline S78 degree 3 poles (30.1223, 20.9189) (30.0655, 20.8002) (29.9428, 20.5438) (29.7104, 20.3787) (29.5857, 20.29) knots 0 0 0 0 0.038855 0.08389 0.08389 0.08389 0.08389
  spline S79 degree 3 poles (29.5857, 20.29) (29.4346, 20.2113) (29.1149, 20.0447) (28.7541, 20.0285) (28.5637, 20.02) knots 0 0 0 0 0.050469 0.106844 0.106844 0.106844 0.106844
  spline S80 degree 3 poles (28.5637, 20.02) (28.3685, 20.0262) (28.0061, 20.0378) (27.6743, 20.1823) (27.5212, 20.249) knots 0 0 0 0 0.057962 0.107598 0.107598 0.107598 0.107598
  spline S81 degree 3 poles (27.5212, 20.249) (27.3967, 20.3306) (27.1545, 20.4895) (27.0356, 20.7532) (26.9778, 20.8813) knots 0 0 0 0 0.043651 0.084934 0.084934 0.084934 0.084934
  spline S82 degree 3 poles (26.9778, 20.8813) (26.9391, 21.0502) (26.8474, 21.4512) (26.8455, 21.8631) (26.8445, 22.1015) knots 0 0 0 0 0.051816 0.123073 0.123073 0.123073 0.123073
  line L72 (26.8445, 22.1015) -> (26.8445, 23.7182)
  spline S83 degree 3 poles (26.8445, 23.7182) (26.8447, 23.8927) (26.8451, 24.1919) (26.8736, 24.4896) (26.8855, 24.6138) knots 0 0 0 0 0.052305 0.089688 0.089688 0.089688 0.089688
  spline S84 degree 3 poles (26.8855, 24.6138) (26.9069, 24.7144) (26.951, 24.9222) (27.0679, 25.0998) (27.1282, 25.1914) knots 0 0 0 0 0.030577 0.063147 0.063147 0.063147 0.063147
  spline S85 degree 3 poles (27.1282, 25.1914) (27.2048, 25.2795) (27.3635, 25.4619) (27.5802, 25.5697) (27.6921, 25.6255) knots 0 0 0 0 0.034683 0.071791 0.071791 0.071791 0.071791
  spline S86 degree 3 poles (27.6921, 25.6255) (27.8204, 25.6723) (28.0885, 25.7702) (28.3739, 25.7806) (28.5227, 25.7861) knots 0 0 0 0 0.040704 0.085063 0.085063 0.085063 0.085063
  spline S87 degree 3 poles (28.5227, 25.7861) (28.7194, 25.7792) (29.0861, 25.7663) (29.4181, 25.6117) (29.572, 25.54) knots 0 0 0 0 0.058345 0.108757 0.108757 0.108757 0.108757
  spline S88 degree 3 poles (29.572, 25.54) (29.6966, 25.4567) (29.9325, 25.299) (30.0568, 25.0447) (30.1155, 24.9248) knots 0 0 0 0 0.044052 0.0834 0.0834 0.0834 0.0834
  spline S89 degree 3 poles (30.1155, 24.9248) (30.1531, 24.7694) (30.2437, 24.3948) (30.2447, 24.0089) (30.2454, 23.7832) knots 0 0 0 0 0.047829 0.115241 0.115241 0.115241 0.115241
  line L73 (30.2454, 23.7832) -> (30.2454, 23.2568)
  line L74 (34.1897, 25.6699) -> (33.366, 23.1714)
  line L75 (33.366, 23.1714) -> (34.2683, 20.1362)
  line L76 (34.2683, 20.1362) -> (32.7815, 20.1362)
  line L77 (32.7815, 20.1362) -> (32.2004, 22.5083)
  line L78 (32.2004, 22.5083) -> (32.2004, 20.1362)
  line L79 (32.2004, 20.1362) -> (30.7615, 20.1362)
  line L80 (30.7615, 20.1362) -> (30.7615, 25.6699)
  line L81 (30.7615, 25.6699) -> (32.2004, 25.6699)
  line L82 (32.2004, 25.6699) -> (32.2004, 23.52)
  line L83 (32.2004, 23.52) -> (32.8396, 25.6699)
  line L84 (32.8396, 25.6699) -> (34.1897, 25.6699)
  line L85 (35.7517, 25.6699) -> (37.1872, 25.6699)
  spline S90 degree 3 poles (37.1872, 25.6699) (37.3872, 25.6689) (37.734, 25.6673) (38.0727, 25.5947) (38.2161, 25.5639) knots 0 0 0 0 0.059788 0.103665 0.103665 0.103665 0.103665
  spline S91 degree 3 poles (38.2161, 25.5639) (38.3283, 25.5187) (38.5563, 25.4267) (38.7069, 25.2321) (38.7834, 25.1333) knots 0 0 0 0 0.035616 0.072381 0.072381 0.072381 0.072381
  spline S92 degree 3 poles (38.7834, 25.1333) (38.8458, 24.9951) (38.9943, 24.6665) (38.9971, 24.3042) (38.9988, 24.0942) knots 0 0 0 0 0.045036 0.107135 0.107135 0.107135 0.107135
  spline S93 degree 3 poles (38.9988, 24.0942) (38.9984, 23.9537) (38.9977, 23.7151) (38.8895, 23.5042) (38.845, 23.4175) knots 0 0 0 0 0.041366 0.070258 0.070258 0.070258 0.070258
  spline S94 degree 3 poles (38.845, 23.4175) (38.773, 23.3555) (38.6002, 23.2068) (38.377, 23.1542) (38.2468, 23.1235) knots 0 0 0 0 0.02813 0.0675 0.0675 0.0675 0.0675
  spline S95 degree 3 poles (38.2468, 23.1235) (38.3943, 23.0868) (38.6553, 23.0218) (38.8422, 22.8307) (38.9236, 22.7475) knots 0 0 0 0 0.044489 0.078765 0.078765 0.078765 0.078765
  spline S96 degree 3 poles (38.9236, 22.7475) (38.9752, 22.6393) (39.0952, 22.3876) (39.0991, 22.1075) (39.1013, 21.9477) knots 0 0 0 0 0.035575 0.082782 0.082782 0.082782 0.082782
  line L86 (39.1013, 21.9477) -> (39.1013, 21.435)
  spline S97 degree 3 poles (39.1013, 21.435) (39.1002, 21.2707) (39.0984, 20.9867) (39.0091, 20.7178) (38.9714, 20.6045) knots 0 0 0 0 0.048899 0.084522 0.084522 0.084522 0.084522
  spline S98 degree 3 poles (38.9714, 20.6045) (38.9229, 20.5216) (38.8259, 20.356) (38.6517, 20.2755) (38.5647, 20.2353) knots 0 0 0 0 0.028082 0.056117 0.056117 0.056117 0.056117
  spline S99 degree 3 poles (38.5647, 20.2353) (38.4227, 20.2068) (38.0443, 20.1309) (37.6577, 20.1342) (37.4163, 20.1362) knots 0 0 0 0 0.043367 0.115528 0.115528 0.115528 0.115528
  line L87 (37.4163, 20.1362) -> (35.7517, 20.1362)
  line L88 (35.7517, 20.1362) -> (35.7517, 25.6699)
  line L89 (37.1907, 24.7231) -> (37.1907, 23.4927)
  spline S100 degree 3 poles (37.1907, 23.4927) (37.218, 23.4936) (37.2658, 23.4954) (37.3137, 23.4959) (37.3342, 23.4961) knots 0 0 0 0 0.008207 0.01436 0.01436 0.01436 0.01436
  spline S101 degree 3 poles (37.3342, 23.4961) (37.3956, 23.4964) (37.5002, 23.4971) (37.5738, 23.5689) (37.6042, 23.5986) knots 0 0 0 0 0.017535 0.029879 0.029879 0.029879 0.029879
  spline S102 degree 3 poles (37.6042, 23.5986) (37.6208, 23.6659) (37.6691, 23.8616) (37.665, 24.0639) (37.6623, 24.1968) knots 0 0 0 0 0.020715 0.060305 0.060305 0.060305 0.060305
  spline S103 degree 3 poles (37.6623, 24.1968) (37.6626, 24.2709) (37.663, 24.3941) (37.6283, 24.5121) (37.6145, 24.5591) knots 0 0 0 0 0.022078 0.03671 0.03671 0.03671 0.03671
  spline S104 degree 3 poles (37.6145, 24.5591) (37.5987, 24.5905) (37.5699, 24.6481) (37.5135, 24.6786) (37.488, 24.6924) knots 0 0 0 0 0.010263 0.018771 0.018771 0.018771 0.018771
  spline S105 degree 3 poles (37.488, 24.6924) (37.4508, 24.7005) (37.353, 24.7218) (37.2528, 24.7226) (37.1907, 24.7231) knots 0 0 0 0 0.011396 0.029962 0.029962 0.029962 0.029962
  line L90 (37.1907, 22.6313) -> (37.1907, 21.083)
  spline S106 degree 3 poles (37.1907, 21.083) (37.276, 21.0844) (37.4134, 21.0866) (37.5319, 21.1534) (37.5769, 21.1787) knots 0 0 0 0 0.025035 0.040322 0.040322 0.040322 0.040322
  spline S107 degree 3 poles (37.5769, 21.1787) (37.6014, 21.2272) (37.6676, 21.3579) (37.6644, 21.506) (37.6623, 21.5991) knots 0 0 0 0 0.016112 0.043454 0.043454 0.043454 0.043454
  line L91 (37.6623, 21.5991) -> (37.6623, 22.1152)
  spline S108 degree 3 poles (37.6623, 22.1152) (37.6652, 22.2124) (37.6697, 22.3625) (37.6087, 22.4981) (37.5871, 22.5459) knots 0 0 0 0 0.028602 0.044185 0.044185 0.044185 0.044185
  spline S109 degree 3 poles (37.5871, 22.5459) (37.5423, 22.5682) (37.4187, 22.6296) (37.2794, 22.6307) (37.1907, 22.6313) knots 0 0 0 0 0.014889 0.041 0.041 0.041 0.041
  line L92 (39.6174, 25.6699) -> (42.0168, 25.6699)
  line L93 (42.0168, 25.6699) -> (42.0168, 24.5625)
  line L94 (42.0168, 24.5625) -> (41.0564, 24.5625)
  line L95 (41.0564, 24.5625) -> (41.0564, 23.5132)
  line L96 (41.0564, 23.5132) -> (41.9553, 23.5132)
  line L97 (41.9553, 23.5132) -> (41.9553, 22.4604)
  line L98 (41.9553, 22.4604) -> (41.0564, 22.4604)
  line L99 (41.0564, 22.4604) -> (41.0564, 21.2436)
  line L100 (41.0564, 21.2436) -> (42.1125, 21.2436)
  line L101 (42.1125, 21.2436) -> (42.1125, 20.1362)
  line L102 (42.1125, 20.1362) -> (39.6174, 20.1362)
  line L103 (39.6174, 20.1362) -> (39.6174, 25.6699)
  line L104 (43.9651, 25.6699) -> (43.9651, 21.2436)
  line L105 (43.9651, 21.2436) -> (44.8401, 21.2436)
  line L106 (44.8401, 21.2436) -> (44.8401, 20.1362)
  line L107 (44.8401, 20.1362) -> (42.5261, 20.1362)
  line L108 (42.5261, 20.1362) -> (42.5261, 25.6699)
  line L109 (42.5261, 25.6699) -> (43.9651, 25.6699)
  line L110 (48.0871, 25.6699) -> (48.0871, 24.5625)
  line L111 (48.0871, 24.5625) -> (47.2327, 24.5625)
  line L112 (47.2327, 24.5625) -> (47.2327, 20.1362)
  line L113 (47.2327, 20.1362) -> (45.7937, 20.1362)
  line L114 (45.7937, 20.1362) -> (45.7937, 24.5625)
  line L115 (45.7937, 24.5625) -> (44.9426, 24.5625)
  line L116 (44.9426, 24.5625) -> (44.9426, 25.6699)
  line L117 (44.9426, 25.6699) -> (48.0871, 25.6699)
extrude "押し出し15'" add sketch "スケッチ15 (2)" along normal blind 0.95 separate body contours L0 S0 S1 S2 S3 S4 S5 S6 S7 L1 L2 L3 S8 S9 L4 L5 L6 makes body 33 in component "CASE_LID_print"
extrude "押し出し16'" add sketch "スケッチ15 (2)" along normal blind 0.95 separate body contours L7 S10 S11 L8 S12 S13 makes body 34 in component "CASE_LID_print"
extrude "押し出し17'" add sketch "スケッチ15 (2)" along normal blind 0.95 separate body contours L50 L51 L52 L53 L54 L55 L56 L57 L58 L59 L60 L61 makes body 35 in component "CASE_LID_print"
extrude "押し出し18'" add sketch "スケッチ15 (2)" along normal blind 0.95 separate body contours S61 S62 S63 S64 L64 S65 S66 S67 S68 L65 makes body 36 in component "CASE_LID_print"
extrude "押し出し19" add sketch "スケッチ15 (2)" along normal blind 0.95 separate body contours S45 S46 S47 S48 S49 S50 S51 S52 L62 S53 S54 S55 S56 S57 S58 S59 S60 L63 makes body 37 in component "CASE_LID_print"
extrude "押し出し20" add sketch "スケッチ15 (2)" along normal blind 0.95 separate body contours L44 L45 S16 S17 S18 S19 S20 S21 S22 S23 S24 S25 S26 S27 S28 S29 L46 L47 L48 S30 S31 S32 S33 S34 S35 S36 S37 S38 S39 S40 S41 S42 S43 S44 L49 makes body 38 in component "CASE_LID_print"
extrude "押し出し21" add sketch "スケッチ15 (2)" along normal blind 0.95 separate body contours L66 L67 S69 S70 S71 S72 L68 S73 S74 S75 S76 L69 L70 L71 S77 S78 S79 S80 S81 S82 L72 S83 S84 S85 S86 S87 S88 S89 L73 makes body 39 in component "CASE_LID_print"
extrude "押し出し22" add sketch "スケッチ15 (2)" along normal blind 0.95 separate body contours L38 L39 L40 L41 L42 L43 makes body 40 in component "CASE_LID_print"
extrude "押し出し23" add sketch "スケッチ15 (2)" along normal blind 0.95 separate body contours L74 L75 L76 L77 L78 L79 L80 L81 L82 L83 L84 makes body 41 in component "CASE_LID_print"
extrude "押し出し24" add sketch "スケッチ15 (2)" along normal blind 0.95 separate body contours L29 L30 L31 L32 L33 L34 L35 L36 makes body 42 in component "CASE_LID_print"
extrude "押し出し25" add sketch "スケッチ15 (2)" along normal blind 0.95 separate body contours S14 S15 L37 makes body 43 in component "CASE_LID_print"
extrude "押し出し26" add sketch "スケッチ15 (2)" along normal blind 0.95 separate body contours L90 S106 S107 L91 S108 S109 makes body 44 in component "CASE_LID_print"
extrude "押し出し27" add sketch "スケッチ15 (2)" along normal blind 0.95 separate body contours L89 S100 S101 S102 S103 S104 S105 makes body 45 in component "CASE_LID_print"
extrude "押し出し28" add sketch "スケッチ15 (2)" along normal blind 0.95 separate body contours L85 S90 S91 S92 S93 S94 S95 S96 L86 S97 S98 S99 L87 L88 makes body 46 in component "CASE_LID_print"
extrude "押し出し29" add sketch "スケッチ15 (2)" along normal blind 0.95 separate body contours L25 L26 L27 L28 makes body 47 in component "CASE_LID_print"
extrude "押し出し30" add sketch "スケッチ15 (2)" along normal blind 0.95 separate body contours L92 L93 L94 L95 L96 L97 L98 L99 L100 L101 L102 L103 makes body 48 in component "CASE_LID_print"
extrude "押し出し31" add sketch "スケッチ15 (2)" along normal blind 0.95 separate body contours L21 L22 L23 L24 makes body 49 in component "CASE_LID_print"
extrude "押し出し32" add sketch "スケッチ15 (2)" along normal blind 0.95 separate body contours L104 L105 L106 L107 L108 L109 makes body 50 in component "CASE_LID_print"
extrude "押し出し33" add sketch "スケッチ15 (2)" along normal blind 0.95 separate body contours L9 L10 L11 L12 L13 L14 L15 L16 L17 L18 L19 L20 makes body 51 in component "CASE_LID_print"
extrude "押し出し34" add sketch "スケッチ15 (2)" along normal blind 0.95 separate body contours L110 L111 L112 L113 L114 L115 L116 L117 makes body 52 in component "CASE_LID_print"
move_body "移動1'" bodies 33 34 35 36 37 38 39 40 41 42 43 44 45 46 47 48 49 50 51 52 to x (1, 0, 0) y (0, 1, 0) z (0, 0, 1) at (-24.0486, 0.4969, 0) in component "CASE_LID_print"
combine "結合7'" operation add target body 19 tool bodies 33 34 35 36 37 38 39 40 41 42 43 44 45 46 47 48 49 50 51 52 in component "CASE_LID_print"
ref_plane "作業平面16" through (0, 0, 38.45) normal (0, 0, 1) x (1, 0, 0) in component "CASE_LID_print"
sketch "スケッチ16 (2)" plane through (0, 0, 38.45) normal (0, 0, 1) x (1, 0, 0) in component "CASE_LID_print"
  line L0 (-40, -37) -> (40, -37)
  line L1 (40, -37) -> (45, -32)
  line L2 (45, -32) -> (45, 32)
  line L3 (45, 32) -> (40, 37)
  line L4 (40, 37) -> (-40, 37)
  line L5 (-40, 37) -> (-45, 32)
  line L6 (-45, 32) -> (-45, -32)
  line L7 (-45, -32) -> (-40, -37)
extrude "押し出し35" add sketch "スケッチ16 (2)" along normal blind 2.1 separate body makes body 53 in component "CASE_LID_print"
ref_plane "作業平面17" through (0, 0, 38.25) normal (0, 0, 1) x (1, 0, 0) in component "CASE_LID_print"
sketch "スケッチ17 (2)" plane through (0, 0, 38.25) normal (0, 0, 1) x (1, 0, 0) in component "CASE_LID_print"
  line L0 (-40, -35.6) -> (40, -35.6)
  line L1 (40, -35.6) -> (43.6, -32)
  line L2 (43.6, -32) -> (43.6, 32)
  line L3 (43.6, 32) -> (40, 35.6)
  line L4 (40, 35.6) -> (-40, 35.6)
  line L5 (-40, 35.6) -> (-43.6, 32)
  line L6 (-43.6, 32) -> (-43.6, -32)
  line L7 (-43.6, -32) -> (-40, -35.6)
extrude "押し出し36" add sketch "スケッチ17 (2)" along normal blind 2.5 separate body makes body 54 in component "CASE_LID_print"
combine "結合8'" operation cut target body 53 tool bodies 54 in component "CASE_LID_print"
combine "結合9'" operation cut target body 19 tool bodies 53 in component "CASE_LID_print"
ref_plane "作業平面18" through (0, 0, 39.9) normal (0, 0, 1) x (1, 0, 0) in component "CASE_LID_print"
sketch "スケッチ18 (2)" plane through (0, 0, 39.9) normal (0, 0, 1) x (1, 0, 0) in component "CASE_LID_print"
  circle A0 centre (6, -18) radius 16
extrude "押し出し37" add sketch "スケッチ18 (2)" along normal blind 0.85 separate body makes body 55 in component "CASE_LID_print"
ref_plane "作業平面19" through (0, 0, 39.8) normal (0, 0, 1) x (1, 0, 0) in component "CASE_LID_print"
sketch "スケッチ19" plane through (0, 0, 39.8) normal (0, 0, 1) x (1, 0, 0) in component "CASE_LID_print"
  circle A0 centre (6, -18) radius 10.25
extrude "押し出し38" add sketch "スケッチ19" along normal blind 1.15 separate body makes body 56 in component "CASE_LID_print"
combine "結合10'" operation cut target body 55 tool bodies 56 in component "CASE_LID_print"
combine "結合11'" operation add target body 19 tool bodies 55 in component "CASE_LID_print"
ref_plane "作業平面20" through (0, 0, 39.9) normal (0, 0, 1) x (1, 0, 0) in component "CASE_LID_print"